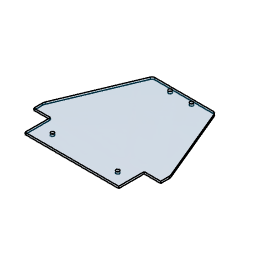
Top Plate v50 (Autodesk Fusion 360 design; units mm, degrees)
Autodesk Fusion 360 part; units mm, degrees
note: some values were not read from the file. Set by a fixed rule: which sketch regions a step uses.
sketch "Main" plane through (0, 0, 0) normal (0, 0, 1) x (1, 0, 0)
  line L0 (17, 0) -> (113, 0)
  line L1 (0, 36) -> (33, 115)
  line L2 (33, 115) -> (97, 115)
  line L3 (97, 115) -> (130, 36)
  line L4 (65, 0) -> (65, 115) construction
  line L5 (0, 36) -> (0, 26)
  line L6 (0, 26) -> (17, 26)
  line L7 (17, 26) -> (17, 0)
  line L8 (130, 36) -> (130, 26)
  line L9 (130, 26) -> (113, 26)
  line L10 (113, 26) -> (113, 0)
  dimension "d2" = 64
  dimension "d4" = 115
  dimension "d10" = 36
  dimension "d25" = 130
  dimension "d26" = 17
  dimension "d27" = 17
  dimension "d30" = 10
  constraint horizontal L0
  constraint parallel L0 L2
  constraint midpoint L0 L4.start
  constraint perpendicular L0 L4
  constraint midpoint L2 L4.end
  constraint vertical L5
  constraint perpendicular L5 L6
  constraint coincident L0 L7.end
  constraint perpendicular L0 L7
  constraint parallel L4 L8
  constraint perpendicular L8 L9
  constraint coincident L0 L10.end
  constraint perpendicular L0 L10
  constraint coincident L0.end L10.end
  constraint vertical origin L5.end
  constraint coincident L0.start L7.end
  constraint horizontal origin L0.end
  constraint horizontal L3.end L1.start
  constraint horizontal L5.end L8.end
  measures "d2" distance of L1.end L2.end
  measures "d4" distance of L0 L2
  measures "d10" distance of origin L1.start
  measures "d25" distance of L5 L8
  measures "d26" distance of L8.end L9.end
  measures "d27" distance of L5.end L6.end
  measures "d30" distance of L1.start L5.end
extrude "Extrude1" add sketch "Main" along normal blind 2
sketch "Holes" plane through (0, 0, 2) normal (0, 0, 1) x (-1, 0, 0)
  line L0 (-130, -36) -> (-97, -115)
  line L1 (-97, -115) -> (-33, -115)
  line L2 (-33, -115) -> (0, -36)
  line L3 (-17, 0) -> (-113, 0)
  line L4 (-31.5797, -111.6) -> (-98.4203, -111.6) construction
  circle A0 centre (-54, -111.6) radius 1.75
  circle A1 centre (-76, -111.6) radius 1.75
  line L5 (-65, -115) -> (-65, 0) construction
  line L6 (-17, -13.5) -> (-113, -13.5) construction
  circle A2 centre (-31.55, -13.5) radius 1.75
  circle A3 centre (-98.45, -13.5) radius 1.75
  line L7 (0, -36) -> (0, -26)
  line L8 (0, -26) -> (-17, -26)
  line L9 (-17, -26) -> (-17, 0)
  line L10 (-113, 0) -> (-113, -26)
  line L11 (-113, -26) -> (-130, -26)
  line L12 (-130, -26) -> (-130, -36)
  dimension "d12" = 3.4
  dimension "d13" = 3.5
  dimension "d14" = 3.5
  dimension "d15" = 22
  dimension "d16" = 11
  dimension "d20" = 13.5
  dimension "d21" = 3.5
  dimension "d22" = 3.5
  dimension "d31" = 14.55
  dimension "d32" = 14.55
  constraint coincident L2 L4.start
  constraint coincident L0 L4.end
  constraint horizontal L4
  constraint coincident L4 A0.centre
  constraint coincident L4 A1.centre
  constraint midpoint L1 L5.start
  constraint midpoint L3 L5.end
  constraint perpendicular L5 L6
  constraint coincident L6 A2.centre
  constraint coincident L6 A3.centre
  constraint coincident L6.start L9
  constraint coincident L6.end L10
  measures "d12" distance of L1 L4
  measures "d13" diameter of A0
  measures "d14" diameter of A1
  measures "d15" distance of A0.centre A1.centre
  measures "d16" distance of A0.centre L5
  measures "d20" distance of L3 L6
  measures "d21" diameter of A2
  measures "d22" diameter of A3
  measures "d31" distance of A2.centre L9
  measures "d32" distance of A3.centre L10
extrude "Extrude2" cut sketch "Holes" against normal through all contours A0 | A1 | A2 | A3
fillet "Fillet3" radius 3 2 edges at (33, 115, 1) (97, 115, 1)
fillet "Fillet4" radius 6 2 edges at (0, 36, 1) (130, 36, 1)
